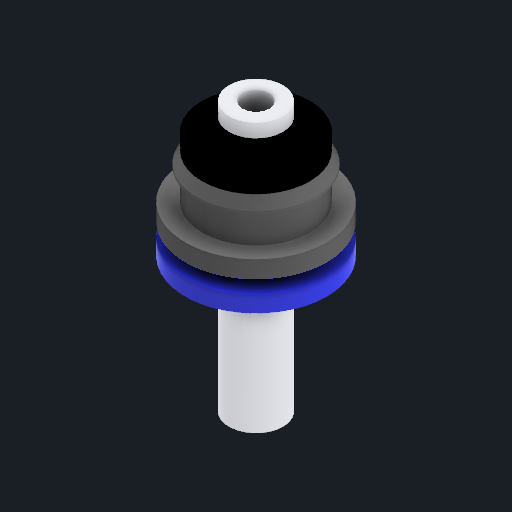
# Autodesk Inventor part: colle ptfe guide
Saved by Autodesk Inventor 2024.3 (Build 283343000, 343)
## iProperties
Created: 2024-09-28
Part Number: colle ptfe guide
Material: Generic
Document SubType Name: Modeling
Designer: MFil
Density: 209.41 g/cm^3
Appearance: Default
Mass: 120 g
Surface Area: 7.92414 cm^2
Volume: 0.573037 cm^3
Author: MFil
Autodesk Inventor part; units mm, degrees
ref_plane "YZ Plane" through (0, 0, 0) normal (1, 0, 0) x (0, 1, 0)
ref_plane "XZ Plane" through (0, 0, 0) normal (0, 1, 0) x (-1, 0, 0)
ref_plane "XY Plane" through (0, 0, 0) normal (0, 0, 1) x (1, 0, 0)
sketch "Sketch1" plane through (0, 0, 0) normal (0, 0, 1) x (1, 0, 0)
  line L0 (0, 0) -> (5.1, 0)
  line L1 (5.1, 0) -> (5.1, 1)
  line L2 (5.1, 1) -> (0, 1)
  line L3 (0, 1) -> (0, 0)
  line L4 (2.55, 1) -> (2.55, -8)
  line L5 (2.55, 1) -> (4.55, 1)
  line L6 (4.55, 1) -> (4.55, 2)
  line L7 (4.55, 2) -> (2.55, 2)
  line L8 (2.55, 2) -> (2.55, 1)
  line L9 (2.55, 0) -> (6.55, 0)
  line L10 (6.55, 0) -> (6.55, -4.5)
  line L11 (6.55, -4.5) -> (2.55, -4.5)
  line L12 (2.55, -4.5) -> (2.55, 0)
  line L13 (6.55, -2.2) -> (6.95, -2.2)
  line L14 (6.95, -2.2) -> (6.95, -1.2)
  line L15 (6.95, -1.2) -> (6.55, -1.2) construction
  line L16 (6.55, -1.2) -> (6.55, -2.2)
  line L17 (6.95, -2.2) -> (6.95, -2)
  line L18 (6.95, -2) -> (6.55, -1.2)
  line L19 (2.55, -4.5) -> (7.8, -4.5)
  line L20 (7.8, -4.5) -> (7.8, -5.8)
  line L21 (7.8, -5.8) -> (2.55, -5.8)
  line L22 (2.55, -5.8) -> (2.55, -4.5)
  line L23 (2.55, -8) -> (7.8, -8)
  line L24 (7.8, -8) -> (7.8, -6.8)
  line L25 (7.8, -6.8) -> (2.55, -6.8)
  line L26 (2.55, -6.8) -> (2.55, -8)
  line L27 (2.55, -5.8) -> (5.55, -5.8)
  line L28 (5.55, -5.8) -> (5.55, -6.8)
  line L29 (5.55, -6.8) -> (2.55, -6.8)
  line L30 (2.55, -6.8) -> (2.55, -5.8)
  line L31 (2.55, -8) -> (4.55, -8)
  line L32 (4.55, -8) -> (4.55, -18)
  line L33 (4.55, -18) -> (2.55, -18)
  line L34 (2.55, -18) -> (2.55, -8)
  line L35 (2.55, 2) -> (3.55, 2)
  line L36 (3.55, 2) -> (3.55, -18)
  line L37 (3.55, -18) -> (2.55, -18)
  line L38 (2.55, -18) -> (2.55, 2)
  dimension "d0" = 5.1
  dimension "d1" = 1
  dimension "d2" = 9
  dimension "d3" = 2
  dimension "d4" = 1
  dimension "d5" = 4
  dimension "d6" = 4.5
  dimension "d7" = 0.4
  dimension "d8" = 1
  dimension "d9" = 0.2
  dimension "d10" = 1.2
  dimension "d11" = 5.25
  dimension "d12" = 1.3
  dimension "d13" = 1.2
  dimension "d14" = 3
  dimension "d15" = 2
  dimension "d16" = 10
  dimension "d17" = 1
  constraints: 78 end point, 18 parallel, 10 perpendicular, 9 horizontal, 5 point on line, 3 midpoint
  measures "d0" distance of L2.end L1.end
  measures "d1" distance of L1.end L0.end
  measures "d2" distance of L4.start L4.end
  measures "d3" distance of L7.end L6.end
  measures "d4" distance of L6.end L5.end
  measures "d5" distance of L10.end L11.end
  measures "d6" distance of L9.end L10.end
  measures "d7" distance of L15.end L14.end
  measures "d8" distance of L14.end L13.end
  measures "d9" distance of L13.end L17.end
  measures "d10" distance between parallel lines of L9 L15
  measures "d11" distance of L20.end L21.end
  measures "d12" distance of L19.end L20.end
  measures "d13" distance of L24.end L23.end
  measures "d14" distance of L28.end L29.end
  measures "d15" distance of L32.end L33.end
  measures "d16" distance of L31.end L32.end
  measures "d17" distance of L36.end L37.end
revolve "Revolution1" add sketch "Sketch1" angle 360 about axis through (2.55, -18, 0) along (0, 1, 0) contours L36 L2 L1 L0 | L0 L9 L10 L11 L36 | L36 L7 L6 L2 | L11 L19 L20 L21 L36 | L21 L28 L25 L36 | L18 L14 L13 L10 | L25 L24 L23 L36 | L23 L32 L33 L36
body "Solid1"
